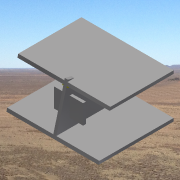
# Autodesk Inventor part: 2p1rim1
Saved by Autodesk Inventor 2014 SP1 (Build 180222100, 222)
## iProperties
Company: HERA Project
Created: 2013-12-03
Part Number: 2p1rim1
Material: Steel, Galvanized
Document SubType Name: Modeling
Designer: David DeBoer
Mass: 492.101 g
Surface Area: 430.611 cm^2
Volume: 62.688 cm^3
Density: 7.85 g/cm^3
Description: end horizontal rim holder 1
Appearance: Galvanized
d0: 3.500 in
d2: 0.120 in
d17: 0.120 in
d18: 3.000 in
d19: 0.00 deg
d20: 15.00 deg
d21: -0.500 in
d22: 1.000 in
d23: 0.00 deg
d24: 0.050 in
d25: 0.050 in
d26: 0.005 in
d27: 0.050 in
d28: 0.170 in
d29: 0.00 deg
d30: 0.00 deg
d31: 0.500 in
d32: 0.00 deg
Author: David DeBoer
Autodesk Inventor part; units mm, degrees
ref_plane "YZ Plane" through (0, 0, 0) normal (1, 0, 0) x (0, 1, 0)
ref_plane "XZ Plane" through (0, 0, 0) normal (0, 1, 0) x (-1, 0, 0)
sketch "Sketch1" plane through (0, 0, 0) normal (0, 0, 1) x (1, 0, 0)
  line L0 (0, 41.148) -> (91.948, 41.148)
  line L1 (91.948, -3.048) -> (0, -3.048)
  line L2 (0, 38.1) -> (0, 41.148)
  line L3 (0, 0) -> (0, -3.048)
  line L4 (88.9, 38.1) -> (91.948, 38.1)
  line L5 (88.9, 0) -> (91.948, 0)
  line L6 (91.948, 38.1) -> (91.948, 41.148)
  line L7 (91.948, 0) -> (91.948, -3.048)
  line L8 (45.974, 38.1) -> (45.974, 0)
  line L9 (49.022, 38.1) -> (49.022, 0)
  line L10 (88.9, 38.1) -> (49.022, 38.1)
  line L11 (45.974, 38.1) -> (0, 38.1)
  line L12 (0, 0) -> (45.974, 0)
  line L13 (49.022, 0) -> (88.9, 0)
  dimension "d0" = 88.9
  dimension "d17" = 3.048
  constraints: 28 end point, 6 parallel, 4 perpendicular, 2 collinear, 2 horizontal
  measures "d0" distance of L3.start L5.start
  measures "d17" distance between parallel lines of L9 L8
extrude "Extrusion6" add sketch "Sketch1" along normal blind 76.2
ref_plane "Work Plane4" through (91.948, 37.861, 63.9327) normal (0, 0.258819, 0.9659258) x (-1, 0, 0)
ref_plane "Work Plane3" through (91.948, 41.148, 76.2) normal (0, 0.258819, 0.9659258) x (-1, 0, 0)
sketch "Sketch6" plane through (91.948, 37.861, 63.9327) normal (0, 0.258819, 0.9659258) x (-1, 0, 0)
  line L0 (-2.4638, -7.3313) -> (94.6916, -7.3313)
  line L1 (94.6916, -7.3313) -> (94.6916, 43.8286)
  line L2 (94.6916, 43.8286) -> (-2.4638, 43.8286)
  line L3 (-2.4638, 43.8286) -> (-2.4638, -7.3313)
  point P0 (91.948, 20.0239)
  constraints: 8 end point, 2 parallel, 1 horizontal, 1 perpendicular
extrude "Extrusion7" cut sketch "Sketch6" along normal blind 25.4
sketch "Sketch7" plane through (45.974, 0, 0) normal (-1, 0, 0) x (0, 0, 1)
  line L0 (0, 38.1) -> (63.8687, 38.1) projected
  line L1 (62.4717, 38.1) -> (63.7417, 38.1)
  line L2 (63.7417, 38.1) -> (63.7417, 36.83)
  line L3 (63.7417, 36.83) -> (62.4717, 36.83)
  line L4 (62.4717, 36.83) -> (62.4717, 38.1)
  dimension "d24" = 1.27
  dimension "d25" = 1.27
  dimension "d26" = 0.127
  constraints: 8 end point, 2 parallel, 1 horizontal, 1 perpendicular, 1 point on line
  measures "d24" distance of L2.end L3.end
  measures "d25" distance of L1.end L2.end
  measures "d26" distance of L0.end L1.end
extrude "Extrusion8" add sketch "Sketch7" along normal blind 1.27 and the other way blind 4.318
sketch "Sketch8" plane through (91.948, 37.861, 63.9327) normal (0, 0.258819, 0.9659258) x (1, 0, 0)
  line L0 (-91.948, 3.403) -> (0, 3.403) projected
  line L1 (-45.974, 3.403) -> (-42.926, 3.403)
  line L2 (-42.926, 3.403) -> (-42.926, 5.2369)
  line L3 (-42.926, 5.2369) -> (-45.974, 5.2369)
  line L4 (-45.974, 5.2369) -> (-45.974, 3.403)
  point P0 (-91.948, -20.0239)
  constraints: 8 end point, 2 parallel, 1 horizontal, 1 midpoint, 1 perpendicular
extrude "Extrusion9" add sketch "Sketch8" against normal blind 12.7
sketch "Sketch10" plane through (45.974, 0, 0) normal (-1, 0, 0) x (0, 0, 1)
  line L0 (58.1292, 9.2578) -> (60.6692, 9.2578)
  line L1 (60.6692, 9.2578) -> (60.6692, 28.3078)
  line L2 (60.6692, 28.3078) -> (58.1292, 28.3078)
  line L3 (58.1292, 28.3078) -> (58.1292, 9.2578)
  dimension "d40" = 2.54
  dimension "d41" = 19.05
  constraints: 8 end point, 2 parallel, 1 horizontal, 1 perpendicular
  measures "d40" distance of L2.end L1.end
  measures "d41" distance of L1.end L0.end
extrude "Extrusion11" add sketch "Sketch10" along normal blind 12.7 and the other way blind 16.51 draft 0.62
body "Solid2"
